Autodesk Inventor part; units mm, degrees
(part 2 of 2)
  line L232 (126.349, -180.9327) -> (126.349, -181.3526)
  spline S229 degree 2 poles (126.349, -181.3526) (126.2823, -181.3798) (126.0798, -181.4588) (126.0008, -181.481) knots 0 0 0 1 2 2 2
  spline S230 degree 2 poles (126.0008, -181.481) (125.8896, -181.5131) (125.7068, -181.5453) (125.5685, -181.5453) knots 0 0 0 1 2 2 2
  spline S231 degree 2 poles (126.0156, -180.0954) (126.0106, -179.9397) (125.9464, -179.7125) (125.8847, -179.6359) knots 0 0 0 1 2 2 2
  spline S232 degree 2 poles (125.8847, -179.6359) (125.818, -179.5495) (125.608, -179.4581) (125.4524, -179.4581) knots 0 0 0 1 2 2 2
  spline S233 degree 2 poles (125.4524, -179.4581) (125.2993, -179.4581) (125.0844, -179.5495) (124.9955, -179.6384) knots 0 0 0 1 2 2 2
  spline S234 degree 2 poles (124.9955, -179.6384) (124.909, -179.7298) (124.8201, -179.9496) (124.8077, -180.0954) knots 0 0 0 1 2 2 2
  line L233 (124.8077, -180.0954) -> (126.0156, -180.0954)
  line L234 (125.2524, -178.8233) -> (124.8399, -178.8233)
  line L235 (124.8399, -178.8233) -> (124.8399, -178.4232)
  line L236 (124.8399, -178.4232) -> (125.2524, -178.4232)
  line L237 (125.2524, -178.4232) -> (125.2524, -178.8233)
  line L238 (126.0971, -178.8233) -> (125.6846, -178.8233)
  line L239 (125.6846, -178.8233) -> (125.6846, -178.4232)
  line L240 (125.6846, -178.4232) -> (126.0971, -178.4232)
  line L241 (126.0971, -178.4232) -> (126.0971, -178.8233)
  line L242 (127.174, -181.4934) -> (126.7887, -181.4934)
  line L243 (126.7887, -181.4934) -> (126.7887, -178.3095)
  line L244 (126.7887, -178.3095) -> (127.174, -178.3095)
  line L245 (127.174, -178.3095) -> (127.174, -181.4934)
  spline S235 degree 2 poles (128.7326, -181.5453) (128.1843, -181.5453) (127.5816, -180.9302) (127.5816, -180.3621) knots 0 0 0 1 2 2 2
  spline S236 degree 2 poles (127.5816, -180.3621) (127.5816, -179.8039) (128.167, -179.1419) (128.6387, -179.1419) knots 0 0 0 1 2 2 2
  spline S237 degree 2 poles (128.6387, -179.1419) (128.8512, -179.1419) (129.1797, -179.2654) (129.3007, -179.3963) knots 0 0 0 1 2 2 2
  spline S238 degree 2 poles (129.3007, -179.3963) (129.4242, -179.5273) (129.5551, -179.9052) (129.5551, -180.1793) knots 0 0 0 1 2 2 2
  line L246 (129.5551, -180.1793) -> (129.5551, -180.3893)
  line L247 (129.5551, -180.3893) -> (127.9718, -180.3893)
  spline S239 degree 2 poles (127.9718, -180.3893) (127.9718, -180.787) (128.372, -181.2093) (128.7277, -181.2093) knots 0 0 0 1 2 2 2
  spline S240 degree 2 poles (128.7277, -181.2093) (128.8536, -181.2093) (129.0982, -181.1525) (129.197, -181.1081) knots 0 0 0 1 2 2 2
  spline S241 degree 2 poles (129.197, -181.1081) (129.3007, -181.0587) (129.444, -180.9722) (129.4909, -180.9327) knots 0 0 0 1 2 2 2
  line L248 (129.4909, -180.9327) -> (129.5131, -180.9327)
  line L249 (129.5131, -180.9327) -> (129.5131, -181.3526)
  spline S242 degree 2 poles (129.5131, -181.3526) (129.4464, -181.3798) (129.2439, -181.4588) (129.1649, -181.481) knots 0 0 0 1 2 2 2
  spline S243 degree 2 poles (129.1649, -181.481) (129.0537, -181.5131) (128.8709, -181.5453) (128.7326, -181.5453) knots 0 0 0 1 2 2 2
  spline S244 degree 2 poles (129.1797, -180.0954) (129.1747, -179.9397) (129.1105, -179.7125) (129.0488, -179.6359) knots 0 0 0 1 2 2 2
  spline S245 degree 2 poles (129.0488, -179.6359) (128.9821, -179.5495) (128.7721, -179.4581) (128.6165, -179.4581) knots 0 0 0 1 2 2 2
  spline S246 degree 2 poles (128.6165, -179.4581) (128.4634, -179.4581) (128.2485, -179.5495) (128.1596, -179.6384) knots 0 0 0 1 2 2 2
  spline S247 degree 2 poles (128.1596, -179.6384) (128.0731, -179.7298) (127.9842, -179.9496) (127.9718, -180.0954) knots 0 0 0 1 2 2 2
  line L250 (127.9718, -180.0954) -> (129.1797, -180.0954)
  line L251 (134.7002, -178.4454) -> (133.9345, -181.4934)
  line L252 (133.9345, -181.4934) -> (133.48, -181.4934)
  line L253 (133.48, -181.4934) -> (132.86, -178.9641)
  line L254 (132.86, -178.9641) -> (132.2573, -181.4934)
  line L255 (132.2573, -181.4934) -> (131.8078, -181.4934)
  line L256 (131.8078, -181.4934) -> (131.0297, -178.4454)
  line L257 (131.0297, -178.4454) -> (131.4472, -178.4454)
  line L258 (131.4472, -178.4454) -> (132.0597, -180.9722)
  line L259 (132.0597, -180.9722) -> (132.6673, -178.4454)
  line L260 (132.6673, -178.4454) -> (133.0798, -178.4454)
  line L261 (133.0798, -178.4454) -> (133.6924, -181.0019)
  line L262 (133.6924, -181.0019) -> (134.3025, -178.4454)
  line L263 (134.3025, -178.4454) -> (134.7002, -178.4454)
  spline S248 degree 2 poles (136.0266, -181.5453) (135.4782, -181.5453) (134.8755, -180.9302) (134.8755, -180.3621) knots 0 0 0 1 2 2 2
  spline S249 degree 2 poles (134.8755, -180.3621) (134.8755, -179.8039) (135.4609, -179.1419) (135.9327, -179.1419) knots 0 0 0 1 2 2 2
  spline S250 degree 2 poles (135.9327, -179.1419) (136.1451, -179.1419) (136.4736, -179.2654) (136.5947, -179.3963) knots 0 0 0 1 2 2 2
  spline S251 degree 2 poles (136.5947, -179.3963) (136.7182, -179.5273) (136.8491, -179.9052) (136.8491, -180.1793) knots 0 0 0 1 2 2 2
  line L264 (136.8491, -180.1793) -> (136.8491, -180.3893)
  line L265 (136.8491, -180.3893) -> (135.2658, -180.3893)
  spline S252 degree 2 poles (135.2658, -180.3893) (135.2658, -180.787) (135.6659, -181.2093) (136.0216, -181.2093) knots 0 0 0 1 2 2 2
  spline S253 degree 2 poles (136.0216, -181.2093) (136.1476, -181.2093) (136.3921, -181.1525) (136.4909, -181.1081) knots 0 0 0 1 2 2 2
  spline S254 degree 2 poles (136.4909, -181.1081) (136.5947, -181.0587) (136.7379, -180.9722) (136.7849, -180.9327) knots 0 0 0 1 2 2 2
  line L266 (136.7849, -180.9327) -> (136.8071, -180.9327)
  line L267 (136.8071, -180.9327) -> (136.8071, -181.3526)
  spline S255 degree 2 poles (136.8071, -181.3526) (136.7404, -181.3798) (136.5379, -181.4588) (136.4588, -181.481) knots 0 0 0 1 2 2 2
  spline S256 degree 2 poles (136.4588, -181.481) (136.3477, -181.5131) (136.1649, -181.5453) (136.0266, -181.5453) knots 0 0 0 1 2 2 2
  spline S257 degree 2 poles (136.4736, -180.0954) (136.4687, -179.9397) (136.4045, -179.7125) (136.3427, -179.6359) knots 0 0 0 1 2 2 2
  spline S258 degree 2 poles (136.3427, -179.6359) (136.276, -179.5495) (136.0661, -179.4581) (135.9105, -179.4581) knots 0 0 0 1 2 2 2
  spline S259 degree 2 poles (135.9105, -179.4581) (135.7573, -179.4581) (135.5424, -179.5495) (135.4535, -179.6384) knots 0 0 0 1 2 2 2
  spline S260 degree 2 poles (135.4535, -179.6384) (135.3671, -179.7298) (135.2781, -179.9496) (135.2658, -180.0954) knots 0 0 0 1 2 2 2
  line L268 (135.2658, -180.0954) -> (136.4736, -180.0954)
  spline S261 degree 2 poles (137.9309, -181.5378) (137.6173, -181.5378) (137.264, -181.1797) (137.264, -180.7919) knots 0 0 0 1 2 2 2
  line L269 (137.264, -180.7919) -> (137.264, -179.5248)
  line L270 (137.264, -179.5248) -> (137.0047, -179.5248)
  line L271 (137.0047, -179.5248) -> (137.0047, -179.2062)
  line L272 (137.0047, -179.2062) -> (137.264, -179.2062)
  line L273 (137.264, -179.2062) -> (137.264, -178.5491)
  line L274 (137.264, -178.5491) -> (137.6494, -178.5491)
  line L275 (137.6494, -178.5491) -> (137.6494, -179.2062)
  line L276 (137.6494, -179.2062) -> (138.3583, -179.2062)
  line L277 (138.3583, -179.2062) -> (138.3583, -179.5248)
  line L278 (138.3583, -179.5248) -> (137.6494, -179.5248)
  line L279 (137.6494, -179.5248) -> (137.6494, -180.6141)
  spline S262 degree 2 poles (137.6494, -180.6141) (137.6494, -180.787) (137.6617, -180.9772) (137.7037, -181.0587) knots 0 0 0 1 2 2 2
  spline S263 degree 2 poles (137.7037, -181.0587) (137.7383, -181.1303) (137.8939, -181.2019) (138.0273, -181.2019) knots 0 0 0 1 2 2 2
  spline S264 degree 2 poles (138.0273, -181.2019) (138.1211, -181.2019) (138.2965, -181.1451) (138.336, -181.1278) knots 0 0 0 1 2 2 2
  line L280 (138.336, -181.1278) -> (138.3583, -181.1278)
  line L281 (138.3583, -181.1278) -> (138.3583, -181.4736)
  spline S265 degree 2 poles (138.3583, -181.4736) (138.2496, -181.5033) (138.0273, -181.5378) (137.9309, -181.5378) knots 0 0 0 1 2 2 2
  spline S266 degree 2 poles (139.6353, -181.5453) (139.0869, -181.5453) (138.4842, -180.9302) (138.4842, -180.3621) knots 0 0 0 1 2 2 2
  spline S267 degree 2 poles (138.4842, -180.3621) (138.4842, -179.8039) (139.0696, -179.1419) (139.5414, -179.1419) knots 0 0 0 1 2 2 2
  spline S268 degree 2 poles (139.5414, -179.1419) (139.7538, -179.1419) (140.0823, -179.2654) (140.2034, -179.3963) knots 0 0 0 1 2 2 2
  spline S269 degree 2 poles (140.2034, -179.3963) (140.3269, -179.5273) (140.4578, -179.9052) (140.4578, -180.1793) knots 0 0 0 1 2 2 2
  line L282 (140.4578, -180.1793) -> (140.4578, -180.3893)
  line L283 (140.4578, -180.3893) -> (138.8745, -180.3893)
  spline S270 degree 2 poles (138.8745, -180.3893) (138.8745, -180.787) (139.2746, -181.2093) (139.6303, -181.2093) knots 0 0 0 1 2 2 2
  spline S271 degree 2 poles (139.6303, -181.2093) (139.7563, -181.2093) (140.0008, -181.1525) (140.0996, -181.1081) knots 0 0 0 1 2 2 2
  spline S272 degree 2 poles (140.0996, -181.1081) (140.2034, -181.0587) (140.3466, -180.9722) (140.3935, -180.9327) knots 0 0 0 1 2 2 2
  line L284 (140.3935, -180.9327) -> (140.4158, -180.9327)
  line L285 (140.4158, -180.9327) -> (140.4158, -181.3526)
  spline S273 degree 2 poles (140.4158, -181.3526) (140.3491, -181.3798) (140.1465, -181.4588) (140.0675, -181.481) knots 0 0 0 1 2 2 2
  spline S274 degree 2 poles (140.0675, -181.481) (139.9564, -181.5131) (139.7736, -181.5453) (139.6353, -181.5453) knots 0 0 0 1 2 2 2
  spline S275 degree 2 poles (140.0823, -180.0954) (140.0774, -179.9397) (140.0132, -179.7125) (139.9514, -179.6359) knots 0 0 0 1 2 2 2
  spline S276 degree 2 poles (139.9514, -179.6359) (139.8847, -179.5495) (139.6748, -179.4581) (139.5192, -179.4581) knots 0 0 0 1 2 2 2
  spline S277 degree 2 poles (139.5192, -179.4581) (139.366, -179.4581) (139.1511, -179.5495) (139.0622, -179.6384) knots 0 0 0 1 2 2 2
  spline S278 degree 2 poles (139.0622, -179.6384) (138.9758, -179.7298) (138.8868, -179.9496) (138.8745, -180.0954) knots 0 0 0 1 2 2 2
  line L286 (138.8745, -180.0954) -> (140.0823, -180.0954)
  line L287 (142.6437, -181.4934) -> (142.2584, -181.4934)
  line L288 (142.2584, -181.4934) -> (142.2584, -180.1892)
  spline S279 degree 2 poles (142.2584, -180.1892) (142.2584, -180.0311) (142.2288, -179.7594) (142.1843, -179.6779) knots 0 0 0 1 2 2 2
  spline S280 degree 2 poles (142.1843, -179.6779) (142.1374, -179.5915) (141.9694, -179.5075) (141.8262, -179.5075) knots 0 0 0 1 2 2 2
  spline S281 degree 2 poles (141.8262, -179.5075) (141.6829, -179.5075) (141.3791, -179.6606) (141.2334, -179.7841) knots 0 0 0 1 2 2 2
  line L289 (141.2334, -179.7841) -> (141.2334, -181.4934)
  line L290 (141.2334, -181.4934) -> (140.848, -181.4934)
  line L291 (140.848, -181.4934) -> (140.848, -179.2062)
  line L292 (140.848, -179.2062) -> (141.2334, -179.2062)
  line L293 (141.2334, -179.2062) -> (141.2334, -179.4606)
  spline S282 degree 2 poles (141.2334, -179.4606) (141.4063, -179.305) (141.7397, -179.1419) (141.9274, -179.1419) knots 0 0 0 1 2 2 2
  spline S283 degree 2 poles (141.9274, -179.1419) (142.2634, -179.1419) (142.6437, -179.5865) (142.6437, -180.0089) knots 0 0 0 1 2 2 2
  line L294 (142.6437, -180.0089) -> (142.6437, -181.4934)
  spline S284 degree 2 poles (143.8022, -181.5477) (143.5725, -181.5477) (143.1748, -181.4242) (143.0439, -181.3551) knots 0 0 0 1 2 2 2
  line L295 (143.0439, -181.3551) -> (143.0439, -180.9228)
  line L296 (143.0439, -180.9228) -> (143.0636, -180.9228)
  spline S285 degree 2 poles (143.0636, -180.9228) (143.113, -180.9623) (143.2464, -181.0562) (143.3576, -181.1081) knots 0 0 0 1 2 2 2
  spline S286 degree 2 poles (143.3576, -181.1081) (143.4539, -181.155) (143.691, -181.2242) (143.817, -181.2242) knots 0 0 0 1 2 2 2
  spline S287 degree 2 poles (143.817, -181.2242) (143.9084, -181.2242) (144.1183, -181.1822) (144.1677, -181.1476) knots 0 0 0 1 2 2 2
  spline S288 degree 2 poles (144.1677, -181.1476) (144.2394, -181.1007) (144.3036, -180.9944) (144.3036, -180.8858) knots 0 0 0 1 2 2 2
  spline S289 degree 2 poles (144.3036, -180.8858) (144.3036, -180.7499) (144.1554, -180.6091) (143.9652, -180.5622) knots 0 0 0 1 2 2 2
  spline S290 degree 2 poles (143.9652, -180.5622) (143.8911, -180.5449) (143.654, -180.4955) (143.5527, -180.4683) knots 0 0 0 1 2 2 2
  spline S291 degree 2 poles (143.5527, -180.4683) (143.2909, -180.3918) (143.0538, -180.0756) (143.0538, -179.8508) knots 0 0 0 1 2 2 2
  spline S292 degree 2 poles (143.0538, -179.8508) (143.0538, -179.5396) (143.5206, -179.1518) (143.9059, -179.1518) knots 0 0 0 1 2 2 2
  spline S293 degree 2 poles (143.9059, -179.1518) (144.0961, -179.1518) (144.4814, -179.2457) (144.6123, -179.3173) knots 0 0 0 1 2 2 2
  line L297 (144.6123, -179.3173) -> (144.6123, -179.7298)
  line L298 (144.6123, -179.7298) -> (144.5926, -179.7298)
  spline S294 degree 2 poles (144.5926, -179.7298) (144.4444, -179.6112) (144.0838, -179.4754) (143.8985, -179.4754) knots 0 0 0 1 2 2 2
  spline S295 degree 2 poles (143.8985, -179.4754) (143.7083, -179.4754) (143.4465, -179.6359) (143.4465, -179.7965) knots 0 0 0 1 2 2 2
  spline S296 degree 2 poles (143.4465, -179.7965) (143.4465, -179.9422) (143.6021, -180.083) (143.775, -180.1275) knots 0 0 0 1 2 2 2
  spline S297 degree 2 poles (143.775, -180.1275) (143.859, -180.1497) (144.0714, -180.1942) (144.1875, -180.2213) knots 0 0 0 1 2 2 2
  spline S298 degree 2 poles (144.1875, -180.2213) (144.4394, -180.2856) (144.6963, -180.5795) (144.6963, -180.8339) knots 0 0 0 1 2 2 2
  spline S299 degree 2 poles (144.6963, -180.8339) (144.6963, -180.9821) (144.5802, -181.2439) (144.4666, -181.3402) knots 0 0 0 1 2 2 2
  spline S300 degree 2 poles (144.4666, -181.3402) (144.3456, -181.4415) (144.0368, -181.5477) (143.8022, -181.5477) knots 0 0 0 1 2 2 2
  spline S301 degree 2 poles (145.9634, -181.5453) (145.7263, -181.5453) (145.3336, -181.3995) (145.1928, -181.2513) knots 0 0 0 1 2 2 2
  spline S302 degree 2 poles (145.1928, -181.2513) (145.052, -181.1056) (144.8964, -180.6561) (144.8964, -180.3547) knots 0 0 0 1 2 2 2
  spline S303 degree 2 poles (144.8964, -180.3547) (144.8964, -180.0534) (145.0569, -179.6137) (145.1928, -179.4655) knots 0 0 0 1 2 2 2
  spline S304 degree 2 poles (145.1928, -179.4655) (145.3286, -179.3148) (145.7313, -179.1543) (145.9634, -179.1543) knots 0 0 0 1 2 2 2
  spline S305 degree 2 poles (145.9634, -179.1543) (146.1512, -179.1543) (146.5019, -179.2605) (146.6378, -179.3297) knots 0 0 0 1 2 2 2
  line L299 (146.6378, -179.3297) -> (146.6378, -179.7619)
  line L300 (146.6378, -179.7619) -> (146.6155, -179.7619)
  spline S306 degree 2 poles (146.6155, -179.7619) (146.5735, -179.7273) (146.4451, -179.6384) (146.3537, -179.5915) knots 0 0 0 1 2 2 2
  spline S307 degree 2 poles (146.3537, -179.5915) (146.2722, -179.552) (146.0548, -179.4902) (145.956, -179.4902) knots 0 0 0 1 2 2 2
  spline S308 degree 2 poles (145.956, -179.4902) (145.6572, -179.4902) (145.2941, -179.9422) (145.2941, -180.3547) knots 0 0 0 1 2 2 2
  spline S309 degree 2 poles (145.2941, -180.3547) (145.2941, -180.7573) (145.6448, -181.2093) (145.956, -181.2093) knots 0 0 0 1 2 2 2
  spline S310 degree 2 poles (145.956, -181.2093) (146.1437, -181.2093) (146.4846, -181.0537) (146.6155, -180.9327) knots 0 0 0 1 2 2 2
  line L301 (146.6155, -180.9327) -> (146.6378, -180.9327)
  line L302 (146.6378, -180.9327) -> (146.6378, -181.3649)
  spline S311 degree 2 poles (146.6378, -181.3649) (146.5809, -181.3921) (146.408, -181.4687) (146.3389, -181.486) knots 0 0 0 1 2 2 2
  spline S312 degree 2 poles (146.3389, -181.486) (146.2401, -181.5156) (146.0845, -181.5453) (145.9634, -181.5453) knots 0 0 0 1 2 2 2
  line L303 (148.7842, -181.4934) -> (148.3989, -181.4934)
  line L304 (148.3989, -181.4934) -> (148.3989, -180.1892)
  spline S313 degree 2 poles (148.3989, -180.1892) (148.3989, -180.0311) (148.3692, -179.7594) (148.3248, -179.6779) knots 0 0 0 1 2 2 2
  spline S314 degree 2 poles (148.3248, -179.6779) (148.2778, -179.5915) (148.1099, -179.5075) (147.9666, -179.5075) knots 0 0 0 1 2 2 2
  spline S315 degree 2 poles (147.9666, -179.5075) (147.8234, -179.5075) (147.5195, -179.6606) (147.3738, -179.7841) knots 0 0 0 1 2 2 2
  line L305 (147.3738, -179.7841) -> (147.3738, -181.4934)
  line L306 (147.3738, -181.4934) -> (146.9885, -181.4934)
  line L307 (146.9885, -181.4934) -> (146.9885, -178.3095)
  line L308 (146.9885, -178.3095) -> (147.3738, -178.3095)
  line L309 (147.3738, -178.3095) -> (147.3738, -179.4606)
  spline S316 degree 2 poles (147.3738, -179.4606) (147.5467, -179.305) (147.8802, -179.1419) (148.0679, -179.1419) knots 0 0 0 1 2 2 2
  spline S317 degree 2 poles (148.0679, -179.1419) (148.4038, -179.1419) (148.7842, -179.5865) (148.7842, -180.0089) knots 0 0 0 1 2 2 2
  line L310 (148.7842, -180.0089) -> (148.7842, -181.4934)
  spline S318 degree 2 poles (150.5997, -181.2513) (150.5527, -181.2859) (150.3946, -181.4094) (150.3205, -181.4465) knots 0 0 0 1 2 2 2
  spline S319 degree 2 poles (150.3205, -181.4465) (150.2193, -181.5008) (150.0291, -181.5576) (149.8562, -181.5576) knots 0 0 0 1 2 2 2
  spline S320 degree 2 poles (149.8562, -181.5576) (149.7154, -181.5576) (149.461, -181.4514) (149.3646, -181.3551) knots 0 0 0 1 2 2 2
  spline S321 degree 2 poles (149.3646, -181.3551) (149.2733, -181.2612) (149.1621, -180.9846) (149.1621, -180.8314) knots 0 0 0 1 2 2 2
  spline S322 degree 2 poles (149.1621, -180.8314) (149.1621, -180.5943) (149.3622, -180.2584) (149.5795, -180.162) knots 0 0 0 1 2 2 2
  spline S323 degree 2 poles (149.5795, -180.162) (149.7722, -180.0731) (150.2958, -180.0064) (150.5997, -179.9891) knots 0 0 0 1 2 2 2
  line L311 (150.5997, -179.9891) -> (150.5997, -179.915)
  spline S324 degree 2 poles (150.5997, -179.915) (150.5997, -179.7817) (150.5181, -179.6162) (150.444, -179.5692) knots 0 0 0 1 2 2 2
  spline S325 degree 2 poles (150.444, -179.5692) (150.3699, -179.5223) (150.1575, -179.4927) (150.0439, -179.4927) knots 0 0 0 1 2 2 2
  spline S326 degree 2 poles (150.0439, -179.4927) (149.9105, -179.4927) (149.5499, -179.5717) (149.3696, -179.6483) knots 0 0 0 1 2 2 2
  line L312 (149.3696, -179.6483) -> (149.3474, -179.6483)
  line L313 (149.3474, -179.6483) -> (149.3474, -179.2556)
  spline S327 degree 2 poles (149.3474, -179.2556) (149.4536, -179.2259) (149.8512, -179.1518) (150.0464, -179.1518) knots 0 0 0 1 2 2 2
  spline S328 degree 2 poles (150.0464, -179.1518) (150.2835, -179.1518) (150.6071, -179.2259) (150.7355, -179.3222) knots 0 0 0 1 2 2 2
  spline S329 degree 2 poles (150.7355, -179.3222) (150.8615, -179.4161) (150.985, -179.715) (150.985, -179.9299) knots 0 0 0 1 2 2 2
  line L314 (150.985, -179.9299) -> (150.985, -181.4934)
  line L315 (150.985, -181.4934) -> (150.5997, -181.4934)
  line L316 (150.5997, -181.4934) -> (150.5997, -181.2513)
  line L317 (150.5997, -180.9302) -> (150.5997, -180.2954)
  spline S330 degree 2 poles (150.5997, -180.2954) (150.4613, -180.3078) (150.0439, -180.3498) (149.913, -180.3893) knots 0 0 0 1 2 2 2
  spline S331 degree 2 poles (149.913, -180.3893) (149.7599, -180.4362) (149.5598, -180.6314) (149.5598, -180.8043) knots 0 0 0 1 2 2 2
  spline S332 degree 2 poles (149.5598, -180.8043) (149.5598, -181.0019) (149.7821, -181.2019) (149.9945, -181.2019) knots 0 0 0 1 2 2 2
  spline S333 degree 2 poles (149.9945, -181.2019) (150.1748, -181.2019) (150.4712, -181.0463) (150.5997, -180.9302) knots 0 0 0 1 2 2 2
  spline S334 degree 2 poles (153.4426, -180.288) (153.4426, -180.8611) (152.8968, -181.5378) (152.4793, -181.5378) knots 0 0 0 1 2 2 2
  spline S335 degree 2 poles (152.4793, -181.5378) (152.3089, -181.5378) (152.0471, -181.4588) (151.9112, -181.3773) knots 0 0 0 1 2 2 2
  line L318 (151.9112, -181.3773) -> (151.9112, -182.3357)
  line L319 (151.9112, -182.3357) -> (151.5259, -182.3357)
  line L320 (151.5259, -182.3357) -> (151.5259, -179.2062)
  line L321 (151.5259, -179.2062) -> (151.9112, -179.2062)
  line L322 (151.9112, -179.2062) -> (151.9112, -179.4457)
  spline S336 degree 2 poles (151.9112, -179.4457) (152.0545, -179.3148) (152.4052, -179.1419) (152.6103, -179.1419) knots 0 0 0 1 2 2 2
  spline S337 degree 2 poles (152.6103, -179.1419) (153.003, -179.1419) (153.4426, -179.7644) (153.4426, -180.288) knots 0 0 0 1 2 2 2
  spline S338 degree 2 poles (153.045, -180.3325) (153.045, -179.9397) (152.7955, -179.5075) (152.5164, -179.5075) knots 0 0 0 1 2 2 2
  spline S339 degree 2 poles (152.5164, -179.5075) (152.3534, -179.5075) (152.0471, -179.6532) (151.9112, -179.7668) knots 0 0 0 1 2 2 2
  line L323 (151.9112, -179.7668) -> (151.9112, -181.0661)
  spline S340 degree 2 poles (151.9112, -181.0661) (152.0619, -181.1377) (152.2768, -181.192) (152.4151, -181.192) knots 0 0 0 1 2 2 2
  spline S341 degree 2 poles (152.4151, -181.192) (152.714, -181.192) (153.045, -180.7524) (153.045, -180.3325) knots 0 0 0 1 2 2 2
  spline S342 degree 2 poles (155.7595, -180.288) (155.7595, -180.8611) (155.2136, -181.5378) (154.7962, -181.5378) knots 0 0 0 1 2 2 2
  spline S343 degree 2 poles (154.7962, -181.5378) (154.6258, -181.5378) (154.364, -181.4588) (154.2281, -181.3773) knots 0 0 0 1 2 2 2
  line L324 (154.2281, -181.3773) -> (154.2281, -182.3357)
  line L325 (154.2281, -182.3357) -> (153.8428, -182.3357)
  line L326 (153.8428, -182.3357) -> (153.8428, -179.2062)
  line L327 (153.8428, -179.2062) -> (154.2281, -179.2062)
  line L328 (154.2281, -179.2062) -> (154.2281, -179.4457)
  spline S344 degree 2 poles (154.2281, -179.4457) (154.3714, -179.3148) (154.7221, -179.1419) (154.9271, -179.1419) knots 0 0 0 1 2 2 2
  spline S345 degree 2 poles (154.9271, -179.1419) (155.3199, -179.1419) (155.7595, -179.7644) (155.7595, -180.288) knots 0 0 0 1 2 2 2
  spline S346 degree 2 poles (155.3618, -180.3325) (155.3618, -179.9397) (155.1124, -179.5075) (154.8333, -179.5075) knots 0 0 0 1 2 2 2
  spline S347 degree 2 poles (154.8333, -179.5075) (154.6702, -179.5075) (154.364, -179.6532) (154.2281, -179.7668) knots 0 0 0 1 2 2 2
  line L329 (154.2281, -179.7668) -> (154.2281, -181.0661)
  spline S348 degree 2 poles (154.2281, -181.0661) (154.3788, -181.1377) (154.5937, -181.192) (154.732, -181.192) knots 0 0 0 1 2 2 2
  spline S349 degree 2 poles (154.732, -181.192) (155.0309, -181.192) (155.3618, -180.7524) (155.3618, -180.3325) knots 0 0 0 1 2 2 2
  spline S350 degree 2 poles (157.1526, -181.5453) (156.6043, -181.5453) (156.0016, -180.9302) (156.0016, -180.3621) knots 0 0 0 1 2 2 2
  spline S351 degree 2 poles (156.0016, -180.3621) (156.0016, -179.8039) (156.587, -179.1419) (157.0587, -179.1419) knots 0 0 0 1 2 2 2
  spline S352 degree 2 poles (157.0587, -179.1419) (157.2712, -179.1419) (157.5997, -179.2654) (157.7207, -179.3963) knots 0 0 0 1 2 2 2
  spline S353 degree 2 poles (157.7207, -179.3963) (157.8442, -179.5273) (157.9751, -179.9052) (157.9751, -180.1793) knots 0 0 0 1 2 2 2
  line L330 (157.9751, -180.1793) -> (157.9751, -180.3893)
  line L331 (157.9751, -180.3893) -> (156.3918, -180.3893)
  spline S354 degree 2 poles (156.3918, -180.3893) (156.3918, -180.787) (156.792, -181.2093) (157.1477, -181.2093) knots 0 0 0 1 2 2 2
  spline S355 degree 2 poles (157.1477, -181.2093) (157.2736, -181.2093) (157.5182, -181.1525) (157.617, -181.1081) knots 0 0 0 1 2 2 2
  spline S356 degree 2 poles (157.617, -181.1081) (157.7207, -181.0587) (157.864, -180.9722) (157.9109, -180.9327) knots 0 0 0 1 2 2 2
  line L332 (157.9109, -180.9327) -> (157.9331, -180.9327)
  line L333 (157.9331, -180.9327) -> (157.9331, -181.3526)
  spline S357 degree 2 poles (157.9331, -181.3526) (157.8664, -181.3798) (157.6639, -181.4588) (157.5849, -181.481) knots 0 0 0 1 2 2 2
  spline S358 degree 2 poles (157.5849, -181.481) (157.4737, -181.5131) (157.2909, -181.5453) (157.1526, -181.5453) knots 0 0 0 1 2 2 2
  spline S359 degree 2 poles (157.5997, -180.0954) (157.5947, -179.9397) (157.5305, -179.7125) (157.4688, -179.6359) knots 0 0 0 1 2 2 2
  spline S360 degree 2 poles (157.4688, -179.6359) (157.4021, -179.5495) (157.1921, -179.4581) (157.0365, -179.4581) knots 0 0 0 1 2 2 2
  spline S361 degree 2 poles (157.0365, -179.4581) (156.8834, -179.4581) (156.6685, -179.5495) (156.5796, -179.6384) knots 0 0 0 1 2 2 2
  spline S362 degree 2 poles (156.5796, -179.6384) (156.4931, -179.7298) (156.4042, -179.9496) (156.3918, -180.0954) knots 0 0 0 1 2 2 2
  line L334 (156.3918, -180.0954) -> (157.5997, -180.0954)
  line L335 (160.1611, -181.4934) -> (159.7758, -181.4934)
  line L336 (159.7758, -181.4934) -> (159.7758, -180.1892)
  spline S363 degree 2 poles (159.7758, -180.1892) (159.7758, -180.0311) (159.7461, -179.7594) (159.7017, -179.6779) knots 0 0 0 1 2 2 2
  spline S364 degree 2 poles (159.7017, -179.6779) (159.6547, -179.5915) (159.4868, -179.5075) (159.3435, -179.5075) knots 0 0 0 1 2 2 2
  spline S365 degree 2 poles (159.3435, -179.5075) (159.2003, -179.5075) (158.8964, -179.6606) (158.7507, -179.7841) knots 0 0 0 1 2 2 2
  line L337 (158.7507, -179.7841) -> (158.7507, -181.4934)
  line L338 (158.7507, -181.4934) -> (158.3654, -181.4934)
  line L339 (158.3654, -181.4934) -> (158.3654, -179.2062)
  line L340 (158.3654, -179.2062) -> (158.7507, -179.2062)
  line L341 (158.7507, -179.2062) -> (158.7507, -179.4606)
  spline S366 degree 2 poles (158.7507, -179.4606) (158.9236, -179.305) (159.2571, -179.1419) (159.4448, -179.1419) knots 0 0 0 1 2 2 2
  spline S367 degree 2 poles (159.4448, -179.1419) (159.7807, -179.1419) (160.1611, -179.5865) (160.1611, -180.0089) knots 0 0 0 1 2 2 2
  line L342 (160.1611, -180.0089) -> (160.1611, -181.4934)
  line L343 (161.4084, -181.4934) -> (160.9194, -181.4934)
  line L344 (160.9194, -181.4934) -> (160.9194, -180.9105)
  line L345 (160.9194, -180.9105) -> (161.4084, -180.9105)
  line L346 (161.4084, -180.9105) -> (161.4084, -181.4934)
  line L347 (161.4084, -179.7891) -> (160.9194, -179.7891)
  line L348 (160.9194, -179.7891) -> (160.9194, -179.2062)
  line L349 (160.9194, -179.2062) -> (161.4084, -179.2062)
  line L350 (161.4084, -179.2062) -> (161.4084, -179.7891)
  line L351 (163.5228, -181.4934) -> (163.5228, -178.4454)
  line L352 (163.5228, -178.4454) -> (165.4296, -178.4454)
  line L353 (165.4296, -178.4454) -> (165.4296, -178.806)
  line L354 (165.4296, -178.806) -> (163.9279, -178.806)
  line L355 (163.9279, -178.806) -> (163.9279, -179.6409)
  line L356 (163.9279, -179.6409) -> (165.3284, -179.6409)
  line L357 (165.3284, -179.6409) -> (165.3284, -180.0015)
  line L358 (165.3284, -180.0015) -> (163.9279, -180.0015)
  line L359 (163.9279, -180.0015) -> (163.9279, -181.1328)
  line L360 (163.9279, -181.1328) -> (165.4296, -181.1328)
  line L361 (165.4296, -181.1328) -> (165.4296, -181.4934)
  line L362 (165.4296, -181.4934) -> (163.5228, -181.4934)
  line L363 (167.6403, -181.4934) -> (165.8742, -181.4934)
  line L364 (165.8742, -181.4934) -> (165.8742, -178.4454)
  line L365 (165.8742, -178.4454) -> (166.2793, -178.4454)
  line L366 (166.2793, -178.4454) -> (166.2793, -181.1328)
  line L367 (166.2793, -181.1328) -> (167.6403, -181.1328)
  line L368 (167.6403, -181.1328) -> (167.6403, -181.4934)
  spline S368 degree 2 poles (170.1153, -178.7937) (170.2882, -178.9962) (170.4808, -179.589) (170.4808, -179.9694) knots 0 0 0 1 2 2 2
  spline S369 degree 2 poles (170.4808, -179.9694) (170.4808, -180.3399) (170.2931, -180.9401) (170.1153, -181.1426) knots 0 0 0 1 2 2 2
  spline S370 degree 2 poles (170.1153, -181.1426) (169.9275, -181.3551) (169.4311, -181.5576) (169.1322, -181.5576) knots 0 0 0 1 2 2 2
  spline S371 degree 2 poles (169.1322, -181.5576) (168.8234, -181.5576) (168.3294, -181.3477) (168.1491, -181.1426) knots 0 0 0 1 2 2 2
  spline S372 degree 2 poles (168.1491, -181.1426) (167.9738, -180.9401) (167.786, -180.3448) (167.786, -179.9694) knots 0 0 0 1 2 2 2
  spline S373 degree 2 poles (167.786, -179.9694) (167.786, -179.5865) (167.9762, -179.0036) (168.1516, -178.7937) knots 0 0 0 1 2 2 2
  spline S374 degree 2 poles (168.1516, -178.7937) (168.3294, -178.5911) (168.8259, -178.3812) (169.1322, -178.3812) knots 0 0 0 1 2 2 2
  spline S375 degree 2 poles (169.1322, -178.3812) (169.4434, -178.3812) (169.9424, -178.5985) (170.1153, -178.7937) knots 0 0 0 1 2 2 2
  spline S376 degree 2 poles (170.0584, -179.9694) (170.0584, -179.668) (169.9275, -179.2012) (169.809, -179.0481) knots 0 0 0 1 2 2 2
  spline S377 degree 2 poles (169.809, -179.0481) (169.6879, -178.89) (169.3471, -178.7319) (169.1347, -178.7319) knots 0 0 0 1 2 2 2
  spline S378 degree 2 poles (169.1347, -178.7319) (168.9148, -178.7319) (168.5838, -178.8851) (168.4579, -179.0481) knots 0 0 0 1 2 2 2
  spline S379 degree 2 poles (168.4579, -179.0481) (168.3368, -179.2037) (168.2084, -179.673) (168.2084, -179.9694) knots 0 0 0 1 2 2 2
  spline S380 degree 2 poles (168.2084, -179.9694) (168.2084, -180.5696) (168.7123, -181.2069) (169.1347, -181.2069) knots 0 0 0 1 2 2 2
  spline S381 degree 2 poles (169.1347, -181.2069) (169.557, -181.2069) (170.0584, -180.5696) (170.0584, -179.9694) knots 0 0 0 1 2 2 2
  line L369 (171.9554, -180.3448) -> (170.8019, -180.3448)
  line L370 (170.8019, -180.3448) -> (170.8019, -179.9743)
  line L371 (170.8019, -179.9743) -> (171.9554, -179.9743)
  line L372 (171.9554, -179.9743) -> (171.9554, -180.3448)
  line L373 (173.5091, -181.4934) -> (172.3284, -181.4934)
  line L374 (172.3284, -181.4934) -> (172.3284, -181.1822)
  line L375 (172.3284, -181.1822) -> (172.7162, -181.1822)
  line L376 (172.7162, -181.1822) -> (172.7162, -178.7566)
  line L377 (172.7162, -178.7566) -> (172.3284, -178.7566)
  line L378 (172.3284, -178.7566) -> (172.3284, -178.4454)
  line L379 (172.3284, -178.4454) -> (173.5091, -178.4454)
  line L380 (173.5091, -178.4454) -> (173.5091, -178.7566)
  line L381 (173.5091, -178.7566) -> (173.1213, -178.7566)
  line L382 (173.1213, -178.7566) -> (173.1213, -181.1822)
  line L383 (173.1213, -181.1822) -> (173.5091, -181.1822)
  line L384 (173.5091, -181.1822) -> (173.5091, -181.4934)
  spline S382 degree 2 poles (175.201, -181.5477) (174.9046, -181.5477) (174.4032, -181.3477) (174.2204, -181.1476) knots 0 0 0 1 2 2 2
  spline S383 degree 2 poles (174.2204, -181.1476) (174.0376, -180.95) (173.8376, -180.3572) (173.8376, -179.9719) knots 0 0 0 1 2 2 2
  spline S384 degree 2 poles (173.8376, -179.9719) (173.8376, -179.589) (174.0327, -179.0209) (174.218, -178.811) knots 0 0 0 1 2 2 2
  spline S385 degree 2 poles (174.218, -178.811) (174.4007, -178.6059) (174.8997, -178.391) (175.2084, -178.391) knots 0 0 0 1 2 2 2
  spline S386 degree 2 poles (175.2084, -178.391) (175.3616, -178.391) (175.6308, -178.4355) (175.7444, -178.4701) knots 0 0 0 1 2 2 2
  spline S387 degree 2 poles (175.7444, -178.4701) (175.8432, -178.5022) (176.0482, -178.5936) (176.1495, -178.6479) knots 0 0 0 1 2 2 2
  line L385 (176.1495, -178.6479) -> (176.1495, -179.137)
  line L386 (176.1495, -179.137) -> (176.1174, -179.137)
  spline S388 degree 2 poles (176.1174, -179.137) (176.0631, -179.0876) (175.8951, -178.9493) (175.7741, -178.8826) knots 0 0 0 1 2 2 2
  spline S389 degree 2 poles (175.7741, -178.8826) (175.658, -178.8184) (175.3838, -178.7369) (175.206, -178.7369) knots 0 0 0 1 2 2 2
  spline S390 degree 2 poles (175.206, -178.7369) (175.0108, -178.7369) (174.6626, -178.8974) (174.5316, -179.0505) knots 0 0 0 1 2 2 2
  spline S391 degree 2 poles (174.5316, -179.0505) (174.4032, -179.2062) (174.2599, -179.6779) (174.2599, -179.9719) knots 0 0 0 1 2 2 2
  spline S392 degree 2 poles (174.2599, -179.9719) (174.2599, -180.2856) (174.4106, -180.7376) (174.5415, -180.8932) knots 0 0 0 1 2 2 2
  spline S393 degree 2 poles (174.5415, -180.8932) (174.67, -181.0438) (175.0133, -181.197) (175.206, -181.197) knots 0 0 0 1 2 2 2
  spline S394 degree 2 poles (175.206, -181.197) (175.3813, -181.197) (175.6802, -181.1105) (175.7963, -181.0463) knots 0 0 0 1 2 2 2
  spline S395 degree 2 poles (175.7963, -181.0463) (175.9074, -180.9821) (176.0729, -180.8487) (176.1199, -180.8018) knots 0 0 0 1 2 2 2
  line L387 (176.1199, -180.8018) -> (176.1495, -180.8018)
  line L388 (176.1495, -180.8018) -> (176.1495, -181.2859)
  spline S396 degree 2 poles (176.1495, -181.2859) (176.0482, -181.3328) (175.8704, -181.4193) (175.7444, -181.4588) knots 0 0 0 1 2 2 2
  spline S397 degree 2 poles (175.7444, -181.4588) (175.611, -181.5033) (175.3838, -181.5477) (175.201, -181.5477) knots 0 0 0 1 2 2 2
  line L389 (177.2388, -181.4934) -> (177.2388, -178.806)
  line L390 (177.2388, -178.806) -> (176.2162, -178.806)
  line L391 (176.2162, -178.806) -> (176.2162, -178.4454)
  line L392 (176.2162, -178.4454) -> (178.6665, -178.4454)
  line L393 (178.6665, -178.4454) -> (178.6665, -178.806)
  line L394 (178.6665, -178.806) -> (177.6439, -178.806)
  line L395 (177.6439, -178.806) -> (177.6439, -181.4934)
  line L396 (177.6439, -181.4934) -> (177.2388, -181.4934)
  point P0 (0, 0)
  point P1 (145, -175)
  dimension "d35" = 110
  dimension "d36" = 50
  dimension "d37" = 5
  dimension "d38" = 5
  dimension "d39" = 70
  dimension "d40" = 13.5
  constraints: 28 end point, 6 parallel, 3 perpendicular, 2 horizontal, 2 midpoint, 8 other
  measures "d35" distance of L2.end L3.end
  measures "d36" distance of L1.end L2.end
  measures "d37" distance between parallel lines of L3 L5
  measures "d38" distance between parallel lines of L5 L9
  measures "d39" distance of L13.start L13.end
  measures "d40" distance of L15.end L13.start
extrude "Extrusion2" cut sketch "Sketch2" against normal blind 1
body "Solid1"
